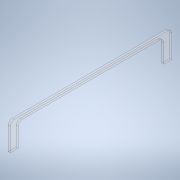
# Autodesk Inventor part: IndexRailOutSides
Saved by Autodesk Inventor 2022 (Build 260153000, 153)
## iProperties
Created: 2022-01-13
Part Number: IndexRailOutSides
Material: Polycarbonate, Clear
Document SubType Name: Modeling
Designer: tagaz
Density: 1.2 g/cm^3
Appearance: Polycarbonate - Clear
Author: tagaz
Autodesk Inventor part; units mm, degrees
ref_plane "YZ Plane" through (0, 0, 0) normal (1, 0, 0) x (0, 1, 0)
ref_plane "XZ Plane" through (0, 0, 0) normal (0, 1, 0) x (-1, 0, 0)
ref_plane "XY Plane" through (0, 0, 0) normal (0, 0, 1) x (1, 0, 0)
sketch "Sketch1" plane through (0, 0, 0) normal (1, 0, 0) x (0, 1, 0)
  line L0 (0, 0) -> (59.309, 0)
  line L1 (84.709, 0) -> (84.709, 12.7)
  line L2 (72.009, 25.4) -> (0, 25.4)
  line L3 (0, 25.4) -> (0, 0)
  line L4 (72.009, -12.7) -> (72.009, -444.5)
  line L5 (84.709, -469.9) -> (84.709, 12.7)
  line L6 (72.009, -482.6) -> (0, -482.6)
  line L7 (0, -482.6) -> (0, -457.2)
  line L8 (0, -457.2) -> (59.309, -457.2)
  arc A0 (84.709, 12.7) -> (72.009, 25.4) centre (72.009, 12.7) ccw
  arc A1 (72.009, -12.7) -> (59.309, 0) centre (59.309, -12.7) ccw
  arc A2 (59.309, -457.2) -> (72.009, -444.5) centre (59.309, -444.5) ccw
  arc A3 (72.009, -482.6) -> (84.709, -469.9) centre (72.009, -469.9) ccw
  dimension "d5" = 25.4
  dimension "d6" = 12.7
  dimension "d7" = 12.7
  dimension "d8" = 12.7
  dimension "d9" = 508
  dimension "d10" = 25.4
  dimension "d11" = 84.709
  dimension "d15" = 84.709
  constraints: 18 end point, 8 point on circle, 8 tangent, 4 centre point, 4 parallel, 2 equal radius, 2 horizontal, 2 perpendicular
  measures "d5" distance of L6.end L7.end
  measures "d6" radius of A0
  measures "d7" radius of A1
  measures "d8" distance between parallel lines of L4 L5
  measures "d9" distance between parallel lines of L2 L6
  measures "d10" distance between parallel lines of L0 L2
  measures "d11" distance between parallel lines of L5 L3
  measures "d15" distance between parallel lines of L5 L7
extrude "Extrusion1" add sketch "Sketch1" along normal blind 6.35
body "Solid1"
